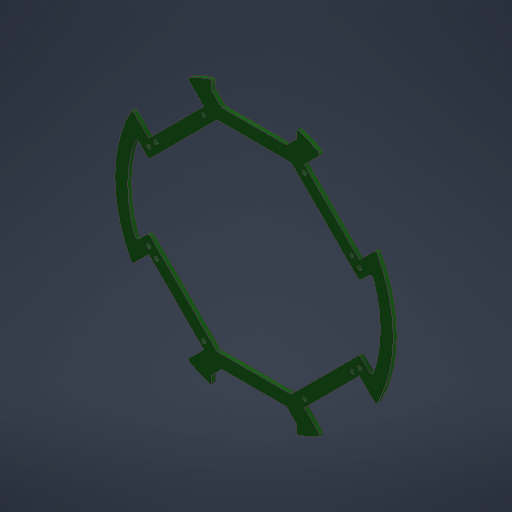
# Autodesk Inventor part: Bottom Ring
Saved by Autodesk Inventor 2026.1 (Build 301233020, 233B)
## iProperties
Created: 2025-10-31
Part Number: Bottom Ring
Material: Generic
Document SubType Name: Modeling
Designer: Bahaa
Density: 1 g/cm^3
Appearance: Default
Author: Bahaa
Autodesk Inventor part; units mm, degrees
ref_plane "YZ Plane" through (0, 0, 0) normal (1, 0, 0) x (0, 1, 0)
ref_plane "XZ Plane" through (0, 0, 0) normal (0, 1, 0) x (-1, 0, 0)
ref_plane "XY Plane" through (0, 0, 0) normal (0, 0, 1) x (1, 0, 0)
sketch "Sketch1" plane through (0, 0, 0) normal (0, 1, 0) x (-1, 0, 0)
  circle A0 centre (0, 0) radius 107.5
  line L0 (107.5, 0) -> (-107.5, 0) construction
  line L1 (-130, -30) -> (-85, -30)
  line L2 (-85, -30) -> (-85, 30)
  line L3 (-85, 30) -> (-130, 30)
  line L4 (-130, 30) -> (-130, -30)
  line L5 (-130, -30) -> (-85, 30) construction
  line L6 (-85, -30) -> (-130, 30) construction
  line L7 (32.5, 102.4695) -> (-32.5, 102.4695)
  line L8 (0, 102.4695) -> (0, 87.4695) construction
  line L9 (-32.5, 117.4695) -> (32.5, 117.4695)
  line L10 (32.5, 117.4695) -> (32.5, 94.9695)
  line L11 (25, 87.4695) -> (-25, 87.4695)
  line L12 (-32.5, 94.9695) -> (-32.5, 117.4695)
  line L13 (-32.5, 117.4695) -> (32.5, 87.4695) construction
  line L14 (32.5, 117.4695) -> (-32.5, 87.4695) construction
  line L15 (-81.3173, -38.8909) -> (-113.1371, -70.7107)
  line L16 (-70.7107, -113.1371) -> (-38.8909, -81.3173)
  line L17 (-70.7107, -113.1371) -> (-81.3173, -38.8909) construction
  line L18 (-113.1371, -70.7107) -> (-70.7107, -113.1371)
  line L19 (-38.8909, -81.3173) -> (-113.1371, -70.7107) construction
  line L20 (-38.8909, -81.3173) -> (-81.3173, -38.8909)
  line L21 (-30, -85) -> (-30, -130)
  line L22 (30, -130) -> (30, -85)
  line L23 (30, -130) -> (-30, -85) construction
  line L24 (-30, -130) -> (30, -130)
  line L25 (30, -85) -> (-30, -130) construction
  line L26 (30, -85) -> (-30, -85)
  line L27 (38.8909, -81.3173) -> (70.7107, -113.1371)
  line L28 (113.1371, -70.7107) -> (81.3173, -38.8909)
  line L29 (113.1371, -70.7107) -> (38.8909, -81.3173) construction
  line L30 (70.7107, -113.1371) -> (113.1371, -70.7107)
  line L31 (81.3173, -38.8909) -> (70.7107, -113.1371) construction
  line L32 (81.3173, -38.8909) -> (38.8909, -81.3173)
  line L33 (85, -30) -> (130, -30)
  line L34 (130, 30) -> (85, 30)
  line L35 (130, 30) -> (85, -30) construction
  line L36 (130, -30) -> (130, 30)
  line L37 (85, 30) -> (130, -30) construction
  line L38 (85, 30) -> (85, -30)
  line L39 (81.3173, 38.8909) -> (113.1371, 70.7107)
  line L40 (70.7107, 113.1371) -> (38.8909, 81.3173)
  line L41 (70.7107, 113.1371) -> (81.3173, 38.8909) construction
  line L42 (113.1371, 70.7107) -> (70.7107, 113.1371)
  line L43 (38.8909, 81.3173) -> (113.1371, 70.7107) construction
  line L44 (38.8909, 81.3173) -> (81.3173, 38.8909)
  line L45 (30, 85) -> (30, 130)
  line L46 (-30, 130) -> (-30, 85)
  line L47 (-30, 130) -> (30, 85) construction
  line L48 (30, 130) -> (-30, 130)
  line L49 (-30, 85) -> (30, 130) construction
  line L50 (-30, 85) -> (30, 85)
  line L51 (-38.8909, 81.3173) -> (-70.7107, 113.1371)
  line L52 (-113.1371, 70.7107) -> (-81.3173, 38.8909)
  line L53 (-113.1371, 70.7107) -> (-38.8909, 81.3173) construction
  line L54 (-70.7107, 113.1371) -> (-113.1371, 70.7107)
  line L55 (-81.3173, 38.8909) -> (-70.7107, 113.1371) construction
  line L56 (-81.3173, 38.8909) -> (-38.8909, 81.3173)
  line L57 (32.5, 94.9695) -> (25, 87.4695)
  line L58 (-25, 87.4695) -> (-32.5, 94.9695)
  line L59 (32.5, -102.4695) -> (-32.5, -102.4695)
  line L60 (0, -102.4695) -> (0, -87.4695) construction
  line L61 (-32.5, -117.4695) -> (32.5, -117.4695)
  line L62 (32.5, -117.4695) -> (32.5, -94.9695)
  line L63 (25, -87.4695) -> (-25, -87.4695)
  line L64 (-32.5, -94.9695) -> (-32.5, -117.4695)
  line L65 (-32.5, -117.4695) -> (32.5, -87.4695) construction
  line L66 (32.5, -117.4695) -> (-32.5, -87.4695) construction
  line L67 (30, -85) -> (30, -130)
  line L68 (-30, -130) -> (-30, -85)
  line L69 (-30, -130) -> (30, -85) construction
  line L70 (30, -130) -> (-30, -130)
  line L71 (-30, -85) -> (30, -130) construction
  line L72 (-30, -85) -> (30, -85)
  line L73 (32.5, -94.9695) -> (25, -87.4695)
  line L74 (-25, -87.4695) -> (-32.5, -94.9695)
  line L75 (-29.1421, 77.4695) -> (-42.5, 90.8274)
  line L76 (-42.5, 90.8274) -> (-42.5, 127.4695)
  line L77 (-42.5, 127.4695) -> (42.5, 127.4695)
  line L78 (42.5, 127.4695) -> (42.5, 90.8274)
  line L79 (42.5, 90.8274) -> (29.1421, 77.4695)
  line L80 (29.1421, 77.4695) -> (-29.1421, 77.4695)
  line L81 (81.3173, 24.7487) -> (24.7487, 81.3173)
  line L82 (24.7487, 81.3173) -> (70.7107, 127.2792)
  line L83 (70.7107, 127.2792) -> (127.2792, 70.7107)
  line L84 (127.2792, 70.7107) -> (81.3173, 24.7487)
  circle A1 centre (0, 0) radius 97.5
  line L85 (24.7487, -81.3173) -> (81.3173, -24.7487)
  line L86 (81.3173, -24.7487) -> (127.2792, -70.7107)
  line L87 (127.2792, -70.7107) -> (70.7107, -127.2792)
  line L88 (70.7107, -127.2792) -> (24.7487, -81.3173)
  line L89 (-81.3173, -24.7487) -> (-24.7487, -81.3173)
  line L90 (-24.7487, -81.3173) -> (-70.7107, -127.2792)
  line L91 (-70.7107, -127.2792) -> (-127.2792, -70.7107)
  line L92 (-127.2792, -70.7107) -> (-81.3173, -24.7487)
  line L93 (-24.7487, 81.3173) -> (-81.3173, 24.7487)
  line L94 (-81.3173, 24.7487) -> (-127.2792, 70.7107)
  line L95 (-127.2792, 70.7107) -> (-70.7107, 127.2792)
  line L96 (-70.7107, 127.2792) -> (-24.7487, 81.3173)
  line L97 (-29.1421, -77.4695) -> (-42.5, -90.8274)
  line L98 (-42.5, -90.8274) -> (-42.5, -127.4695)
  line L99 (-42.5, -127.4695) -> (42.5, -127.4695)
  line L100 (42.5, -127.4695) -> (42.5, -90.8274)
  line L101 (42.5, -90.8274) -> (29.1421, -77.4695)
  line L102 (29.1421, -77.4695) -> (-29.1421, -77.4695)
  line L103 (-85, -30) -> (-85, -26) construction
  line L104 (-85, -26) -> (-81, -26) construction
  circle A2 centre (-81, -26) radius 1.6
  circle A3 centre (-81, 26) radius 1.6
  circle A4 centre (-75.6604, -38.8909) radius 1.6
  circle A5 centre (-38.8909, -75.6604) radius 1.6
  circle A6 centre (-26, -81) radius 1.6
  circle A7 centre (26, -81) radius 1.6
  circle A8 centre (38.8909, -75.6604) radius 1.6
  circle A9 centre (75.6604, -38.8909) radius 1.6
  circle A10 centre (81, -26) radius 1.6
  circle A11 centre (81, 26) radius 1.6
  circle A12 centre (75.6604, 38.8909) radius 1.6
  circle A13 centre (38.8909, 75.6604) radius 1.6
  circle A14 centre (26, 81) radius 1.6
  circle A15 centre (-26, 81) radius 1.6
  circle A16 centre (-38.8909, 75.6604) radius 1.6
  circle A17 centre (-75.6604, 38.8909) radius 1.6
  point P0 (0, 0)
  point P1 (-76.014, -76.014)
  point P2 (0, -107.5)
  point P3 (76.014, -76.014)
  point P4 (107.5, 0)
  point P5 (76.014, 76.014)
  point P6 (0, 107.5)
  point P7 (-76.014, 76.014)
  point P8 (-28.5965, -77.4695)
  point P9 (-91.1582, -34.5896)
  point P10 (-28.5965, 77.4695)
  point P11 (-91.1581, 34.5896)
  point P12 (28.5965, 77.4695)
  point P13 (91.1582, 34.5896)
  point P14 (28.5965, -77.4695)
  point P15 (91.1581, -34.5896)
  point P16 (-32.5, -102.4695)
  point P17 (32.5, -102.4695)
  point P18 (51.7808, -94.2072)
  point P19 (94.2072, -51.7808)
  point P20 (94.2072, 51.7808)
  point P21 (51.7808, 94.2072)
  point P22 (-51.7808, 94.2072)
  point P23 (-94.2072, 51.7808)
  point P24 (-94.2072, -51.7808)
  point P25 (-51.7808, -94.2072)
  point P26 (42.5, 99.0685)
  point P27 (40.406, 88.7333)
  point P28 (-40.406, 88.7333)
  point P29 (34.5896, 91.1581)
  point P30 (40.406, -88.7333)
  point P31 (-34.5896, -91.1581)
  point P32 (-42.5, -99.0685)
  point P33 (-40.406, -88.7333)
  point P34 (42.5, -99.0686)
  point P35 (34.5896, -91.1582)
  point P36 (-42.5, 99.0686)
  point P37 (-34.5896, 91.1582)
  dimension "d48" = 2
  dimension "d0" = 215
  dimension "d4" = 215
  dimension "d14" = 45
  dimension "d15" = 60
  dimension "d21" = 65
  dimension "d22" = 15
  dimension "d23" = 65
  dimension "d24" = 30
  dimension "d27" = 360
  dimension "d29" = 7.5
  dimension "d30" = 7.5
  dimension "d31" = 7.5
  dimension "d32" = 7.5
  dimension "d33" = 10
  dimension "d34" = 10
  dimension "d35" = 10
  dimension "d36" = 10
  dimension "d37" = 10
  dimension "d38" = 10
  dimension "d39" = 10
  dimension "d50" = 4
  dimension "d51" = 4
  dimension "d52" = 3.2
  dimension "d55" = 360
  constraints: 210 end point, 18 centre point, 13 symmetric about line, 9 point on line, 6 midpoint, 6 parallel, 4 horizontal, 4 perpendicular, 4 point on circle, 2 coincident, 1 vertical, 145 other
  measures "d0" diameter of A0
  measures "d4" distance of L0.start L0.end
  measures "d14" distance of L3.end L2.end
  measures "d15" distance of L2.end L1.end
  measures "d21" distance of L7.start L7.end
  measures "d22" distance of L8.start L8.end
  measures "d23" distance of L9.start L9.end
  measures "d24" distance of L14.end L9.start
  measures "d29" distance of L10.end L13.end
  measures "d30" distance of L11.start L13.end
  measures "d31" distance of L11.end L14.end
  measures "d32" distance of L12.start L14.end
  measures "d33" distance between parallel lines of L11 L80
  measures "d34" distance between parallel lines of L44 L81
  measures "d35" radial gap between concentric circles of A0 A1
  measures "d36" distance between parallel lines of L32 L85
  measures "d37" distance between parallel lines of L20 L89
  measures "d38" distance between parallel lines of L56 L93
  measures "d39" distance between parallel lines of L63 L102
  measures "d50" distance of L1.end L103.end
  measures "d51" distance of L103.end L104.end
  measures "d52" diameter of A2
extrude "Extrusion1" add sketch "Sketch1" along normal blind 3 contours A0 L33 A1 L34 | L34 A1 L84 A0 | A0 L86 A1 L33 | L84 A1 L39 A0 | A0 L28 A1 L86 | L84 L34 L38 A11 L81 L80 L79 A1 L40 L44 L39 | L84 L38 L34 | A1 L28 L32 L27 L101 L102 L85 A10 L86 L38 L33 | L33 L38 L86 | L40 A1 L79 L78 A0 | A0 L100 L101 A1 L27 | L78 L79 A1 L82 A0 | L84 L81 A11 | A0 L88 A1 L101 L100 | A10 L85 L86 | L82 A1 L57 L10 A0 | L79 L80 L81 A14 L82 L50 L45 A1 | A0 L62 L73 A1 L88 | A1 L88 L22 L26 A7 L85 L102 L101 | L82 L45 L57 A1 | L80 L93 A15 L96 L50 L82 A14 L81 | A1 L73 L22 L88 | L85 A7 L88 L26 L90 A6 L89 L102 | L82 L50 L96 L46 L58 L11 L57 L45 | L45 L50 L82 | L93 A3 L94 L2 L3 A1 L52 L56 L51 L75 L80 | L80 L75 A1 L96 L46 L50 A15 L93 | A14 L82 L81 | L81 L82 A14 | L88 L26 L22 | L22 L73 L63 L74 L21 L90 L26 L88 | A7 L88 L85 | L85 L88 A7 | L102 L97 A1 L16 L20 L15 L92 L1 L2 A2 L89 | L89 A6 L90 L26 L21 A1 L97 L102 | A15 L96 L93 | L93 L96 A15 | L93 L94 A3 | A2 L92 L89 | A6 L90 L89 | L89 L90 A6 | L12 L58 A1 L96 A0 | L50 L46 L96 | A1 L51 A0 L76 L75 | L75 L76 A0 L96 A1 | A0 L90 A1 L74 L64 | L90 L21 L26 | L97 L98 A0 L16 A1 | A1 L90 A0 L98 L97 | L46 L96 A1 L58 | L94 L3 L2 | L74 A1 L90 L21 | L2 L1 L92 | A1 L94 A0 L52 | L15 A0 L92 A1 | L94 A1 L3 A0 | A1 L1 A0 L3 | A0 L1 A1 L92 picked at (80.9212, 26.6263) picked at (80.9212, -26.6263) picked at (-80.9212, 26.6263) picked at (-80.9212, -26.6263)
fillet "Fillet1" radius 1.5 12 edges at (-32.5, 1.5, 102.4695) (-51.7808, 1.5, 94.2072) (32.5, 1.5, 102.4695) (51.7808, 1.5, 94.2072) (94.2072, 1.5, 51.7808) (94.2072, 1.5, -51.7808) (51.7808, 1.5, -94.2072) (32.5, 1.5, -102.4695) (-32.5, 1.5, -102.4695) (-51.7808, 1.5, -94.2072) (-94.2072, 1.5, -51.7808) (-94.2072, 1.5, 51.7808)
fillet "Fillet2" radius 2 12 edges at (-91.1582, 1.5, 34.5896) (-81.3173, 1.5, 24.7487) (-28.5965, 1.5, 77.4695) (81.3173, 1.5, 24.7487) (91.1581, 1.5, 34.5896) (28.5965, 1.5, 77.4695) (-91.1581, 1.5, -34.5896) (-81.3173, 1.5, -24.7487) (-28.5965, 1.5, -77.4695) (28.5965, 1.5, -77.4695) (91.1582, 1.5, -34.5896) (81.3173, 1.5, -24.7487)
sketch "Sketch2" plane through (0, 0, 0) normal (0, -1, 0) x (1, 0, 0)
  circle A0 centre (38.8909, 75.6604) radius 1.6 projected
  circle A1 centre (75.6604, 38.8909) radius 1.6 projected
  line L0 (75.6604, 38.8909) -> (81.3173, 33.234)
  line L1 (75.6604, 38.8909) -> (83.6604, 38.8909) construction
  circle A2 centre (81.3173, 33.234) radius 1.6
  line L2 (0, 0) -> (0, 47.8849) construction
  circle A3 centre (-81.3173, 33.234) radius 1.6
  line L3 (0, 0) -> (26.8615, 0) construction
  circle A4 centre (81.3173, -33.234) radius 1.6
  circle A5 centre (-81.3173, -33.234) radius 1.6
  dimension "d58" = 8
  dimension "d59" = 45
  dimension "d60" = 3.2
  constraints: 8 end point, 4 centre point, 4 symmetric about line, 2 coincident, 2 horizontal, 1 equal length, 1 vertical, 3 other
  measures "d58" distance of L0.start L0.end
  measures "d59" angle of L0 L1
  measures "d60" diameter of A2
extrude "Extrusion2" cut sketch "Sketch2" against normal through all
equation "\"d4\" = d0"
equation "\"d23\" = d21"
equation "\"d24\" = 2 * d22"
equation "\"d30\" = d29"
equation "\"d32\" = d31"
equation "\"d34\" = d33"
equation "\"d35\" = d33"
equation "\"d36\" = d33"
equation "\"d37\" = d33"
equation "\"d38\" = d33"
equation "\"d39\" = d33"
body "Solid1"
